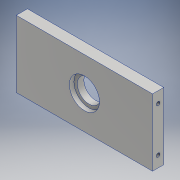
# Autodesk Inventor part: Diffbox_plate_main
Saved by Autodesk Inventor 2018 (Build 220112000, 112)
## iProperties
Created: 2017-10-20
Part Number: Diffbox_plate_main
Material: アルミニウム 6061
Document SubType Name: Modeling
Designer: 翔
Density: 2.7 g/cm^3
Appearance: アルミニウム - フラット
Author: 翔
Autodesk Inventor part; units mm, degrees
ref_plane "YZ Plane" through (0, 0, 0) normal (1, 0, 0) x (0, 1, 0)
ref_plane "XZ Plane" through (0, 0, 0) normal (0, 1, 0) x (-1, 0, 0)
ref_plane "XY Plane" through (0, 0, 0) normal (0, 0, 1) x (1, 0, 0)
sketch "スケッチ1" plane through (0, 0, 0) normal (0, 1, 0) x (-1, 0, 0)
  line L0 (61.0285, -30) -> (-61.0285, -30)
  line L1 (-61.0285, -30) -> (-61.0285, 30)
  line L2 (-61.0285, 30) -> (61.0285, 30)
  line L3 (61.0285, 30) -> (61.0285, -30)
  line L4 (61.0285, -30) -> (-61.0285, 30) construction
  line L5 (-61.0285, -30) -> (61.0285, 30) construction
  point P0 (0, 0)
  dimension "d0" = 60
  dimension "d1" = 122.057
  constraints: 12 end point, 2 midpoint, 2 parallel, 1 horizontal, 1 perpendicular
  measures "d0" distance of L0.end L1.end
  measures "d1" distance of L1.end L2.end
extrude "押し出し1" add sketch "スケッチ1" along normal blind 10
sketch "スケッチ2" plane through (0, 0, 0) normal (0, -1, 0) x (1, 0, 0)
  line L0 (-85.4399, 0) -> (85.4399, 0) projected
  line L1 (0, -42) -> (0, 42) projected
  circle A0 centre (0, 0) radius 13.5
  dimension "d4" = 27
  constraints: 1 centre point, 1 coincident
  measures "d4" diameter of A0
extrude "押し出し2" cut sketch "スケッチ2" against normal blind 4.1
sketch "スケッチ3" plane through (0, 4.1, 0) normal (0, -1, 0) x (1, 0, 0)
  circle A0 centre (0, 0) radius 10.5
  dimension "d7" = 21
  constraints: 1 centre point, 1 coincident
  measures "d7" diameter of A0
extrude "押し出し4" cut sketch "スケッチ3" against normal blind 10
sketch "スケッチ4" plane through (61.0285, 0, 30) normal (1, 0, 0) x (0, 0, -1)
  line L0 (60, 0) -> (0, 0) projected
  line L1 (0, 0) -> (0, 10) projected
  line L2 (60, 0) -> (60, 10) projected
  point P0 (30, 0)
  point P1 (10, 5)
  point P2 (50, 5)
  dimension "d12" = 5
  dimension "d13" = 10
  dimension "d14" = 10
  dimension "d15" = 5
  measures "d12" distance from line of L0 point (10, 5)
  measures "d13" distance from line of point (10, 5) L1
  measures "d14" distance from line of L2 point (50, 5)
  measures "d15" distance from line of L0 point (50, 5)
hole "穴1" at (61.0285, 5, 20) at (61.0285, 5, -20) direction (-1, 0, 0) diameter 3.242 depth 12 thread size "M4x0.7" class "6H" standard "ISO Metric profile"
sketch "スケッチ5" plane through (-61.0285, 0, -30) normal (-1, 0, 0) x (0, 0, 1)
  line L0 (60, 0) -> (0, 0)
  line L1 (0, 0) -> (0, 10)
  line L2 (60, 0) -> (60, 10)
  point P0 (30, 0)
  point P1 (30, 0)
  point P2 (10, 5)
  point P3 (50, 5)
  dimension "d23" = 5
  dimension "d24" = 10
  dimension "d25" = 10
  dimension "d26" = 5
  constraints: 6 end point
  measures "d23" distance from line of L0 point (10, 5)
  measures "d24" distance from line of point (10, 5) L1
  measures "d25" distance from line of L2 point (50, 5)
  measures "d26" distance from line of L0 point (50, 5)
hole "穴2" at (-61.0285, 5, -20) at (-61.0285, 5, 20) direction (1, 0, 0) diameter 3.242 depth 12 thread size "M4x0.7" class "6H" standard "ISO Metric profile"
